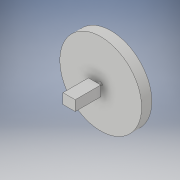
# Autodesk Inventor part: Wheel and Motor
Saved by Autodesk Inventor 2018 (Build 220112000, 112)
## iProperties
Created: 2018-05-15
Part Number: Wheel and Motor
Material: Generic
Document SubType Name: Modeling
Designer: alexs
Density: 1 g/cm^3
Appearance: Default
Author: alexs
Autodesk Inventor part; units mm, degrees
ref_plane "YZ Plane" through (0, 0, 0) normal (1, 0, 0) x (0, 1, 0)
ref_plane "XZ Plane" through (0, 0, 0) normal (0, 1, 0) x (-1, 0, 0)
ref_plane "XY Plane" through (0, 0, 0) normal (0, 0, 1) x (1, 0, 0)
sketch "Sketch1" plane through (0, 0, 0) normal (0, 0, 1) x (1, 0, 0)
  line L0 (0, 0) -> (12, 0)
  line L1 (12, 0) -> (12, 25)
  line L2 (12, 25) -> (0, 25)
  line L3 (0, 25) -> (0, 0)
  dimension "d0" = 12
  dimension "d1" = 25
  constraints: 8 end point, 2 parallel, 1 horizontal, 1 perpendicular
  measures "d0" distance of L2.end L1.end
  measures "d1" distance of L1.end L0.end
extrude "Extrusion1" add sketch "Sketch1" along normal blind 10
sketch "Sketch2" plane through (0, 25, 0) normal (0, 1, 0) x (1, 0, 0)
  line L0 (12, 0) -> (0, 0) construction
  line L1 (0, 0) -> (0, -10) construction
  line L2 (12, -10) -> (0, -10) construction
  line L3 (12, 0) -> (12, -10) construction
  circle A0 centre (6, -5) radius 1.5
  point P0 (12, -5)
  point P1 (6, -10)
  dimension "d4" = 3
  constraints: 2 midpoint, 1 centre point, 1 horizontal alignment, 1 vertical alignment
  measures "d4" diameter of A0
extrude "Extrusion2" add sketch "Sketch2" along normal blind 6
sketch "Sketch3" plane through (6, 31, 5) normal (0, 1, 0) x (1, 0, 0)
  circle A0 centre (0, 0) radius 1.5 construction
  circle A1 centre (0, 0) radius 40
  point P0 (-6, 5)
  dimension "d7" = 80
  constraints: 1 centre point, 1 concentric
  measures "d7" diameter of A1
extrude "Extrusion3" add sketch "Sketch3" along normal blind 10
body "Solid1"
